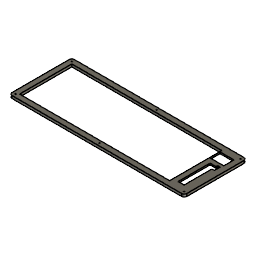
keeb_top (Autodesk Fusion 360 design; units mm, degrees)
part number: 2026-05-28-03-11-49-760
Autodesk Fusion 360 part; units mm, degrees
sketch "Sketch1" plane through (0, 0, 0) normal (0, 0, 1) x (1, 0, 0)
  line L0 (0, 0) -> (336, 0)
  line L1 (336, 0) -> (336, 120)
  line L2 (336, 120) -> (0, 120)
  line L3 (0, 120) -> (0, 0)
  line L4 (10, 110) -> (326, 110)
  line L5 (326, 110) -> (326, 10)
  line L6 (326, 10) -> (10, 10)
  line L7 (10, 10) -> (10, 110)
  line L8 (298, 110) -> (298, 10)
  line L9 (298, 10) -> (326, 10)
  line L10 (326, 10) -> (326, 110)
  line L11 (298.6, 106.03) -> (325.3, 106.03)
  line L12 (325.3, 106.03) -> (325.3, 86.73)
  line L13 (325.3, 86.73) -> (298.6, 86.73)
  line L14 (298.6, 86.73) -> (298.6, 106.03)
  circle A0 centre (6, 114) radius 1
  circle A1 centre (330, 114) radius 1
  circle A2 centre (330, 6) radius 1
  circle A3 centre (6, 6) radius 1
  circle A4 centre (168, 5) radius 1
  circle A5 centre (168, 115) radius 1
  dimension "d1" = 120
  dimension "d2" = 336
  dimension "d3" = 10
  dimension "d4" = 10
  dimension "d5" = 10
  dimension "d6" = 10
  dimension "d7" = 28
  dimension "d8" = 19.3
  dimension "d9" = 0.7
  dimension "d10" = 26.7
  dimension "d11" = 3.97
  dimension "d16" = 2
  dimension "d17" = 6
  dimension "d18" = 6
  dimension "d19" = 2
  dimension "d20" = 6
  dimension "d21" = 6
  dimension "d22" = 2
  dimension "d23" = 6
  dimension "d24" = 6
  dimension "d25" = 2
  dimension "d26" = 6
  dimension "d27" = 6
  dimension "d28" = 2
  dimension "d29" = 168
  dimension "d30" = 2
  dimension "d31" = 168
  constraint horizontal L0
  constraint vertical L1
  constraint horizontal L2
  constraint vertical L3
  constraint coincident L0.start L3.end
  constraint horizontal L4
  constraint vertical L5
  constraint horizontal L6
  constraint vertical L7
  constraint vertical L8
  constraint horizontal L9
  constraint vertical L10
  constraint horizontal L11
  constraint vertical L12
  constraint horizontal L13
  constraint vertical L14
  measures "d1" distance of L0.start L2.end
  measures "d2" distance of L0.start L0.end
  measures "d3" distance of L2 L4
  measures "d4" distance of L1 L5
  measures "d5" distance of L3 L7
  measures "d6" distance of L0 L6
  measures "d7" distance of L8.end L5.end
  measures "d8" distance of L11.start L13.end
  measures "d9" distance of L5 L12
  measures "d10" distance of L11.start L11.end
  measures "d11" distance of L4 L11
  measures "d16" diameter of A0
  measures "d17" distance of L2 A0.centre
  measures "d18" distance of L3 A0.centre
  measures "d19" diameter of A1
  measures "d20" distance of L2 A1.centre
  measures "d21" distance of L1 A1.centre
  measures "d22" diameter of A2
  measures "d23" distance of L1 A2.centre
  measures "d24" distance of L0 A2.centre
  measures "d25" diameter of A3
  measures "d26" distance of L0 A3.centre
  measures "d27" distance of L3 A3.centre
  measures "d28" diameter of A4
  measures "d29" distance of L3 A4.centre
  measures "d30" diameter of A5
  measures "d31" distance of L3 A5.centre
sketch "Sketch4" plane through (0, 0, 0) normal (0, 0, 1) x (1, 0, 0)
  line L0 (319.15, 77.73) -> (307.75, 77.73)
  line L1 (307.75, 77.73) -> (307.75, 16.73)
  line L2 (307.75, 16.73) -> (319.15, 16.73)
  line L3 (319.15, 16.73) -> (319.15, 77.73)
  line L4 (319.15, 77.73) -> (319.15, 80.98)
  line L5 (319.15, 80.98) -> (323.95, 80.98)
  line L6 (323.95, 80.98) -> (323.95, 69.98)
  line L7 (323.95, 69.98) -> (319.15, 69.98)
  line L8 (319.15, 69.98) -> (319.15, 80.98)
  dimension "d50" = 11.4
  dimension "d51" = 61
  dimension "d52" = 3.25
  dimension "d53" = 4.8
  dimension "d54" = 11
  constraint horizontal L0
  constraint vertical L1
  constraint horizontal L2
  constraint vertical L3
  constraint perpendicular L0 L4
  constraint horizontal L5
  constraint vertical L6
  constraint horizontal L7
  constraint vertical L8
  measures "d50" distance of L0.start L0.end
  measures "d51" distance of L0.start L2.end
  measures "d52" distance of L0.start L4.end
  measures "d53" distance of L4.end L5.end
  measures "d54" distance of L4.end L7.end
extrude "Extrude3" add sketch "Sketch1" along normal blind 5 contours L0 L1 L2 L3
extrude "Extrude4" add sketch "Sketch1" along normal blind 5 contours L4 L5 L6 L8 L9 L10
extrude "Extrude5" cut sketch "Sketch1" along normal blind 2 contours L4 L5 L6 L8 L9 L10
extrude "Extrude6" cut sketch "Sketch4" along normal blind 5
fillet "Fillet5" radius 5 1 edges at (336, 0, 2.5)
fillet "Fillet6" radius 5 1 edges at (336, 120, 2.5)
fillet "Fillet7" radius 5 1 edges at (0, 120, 2.5)
fillet "Fillet8" radius 5 1 edges at (0, 0, 2.5)
extrude "Extrude1" [suppressed]
extrude "Extrude2" [suppressed]
fillet "Fillet1" [suppressed]
fillet "Fillet2" [suppressed]
fillet "Fillet3" [suppressed]
fillet "Fillet4" [suppressed]
